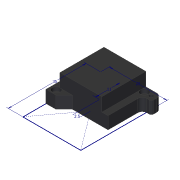
# Autodesk Inventor part: Raman2Go_Adapterplatte2_XY-TischChina
Saved by Autodesk Inventor 2019 (Build 230136000, 136)
## iProperties
Created: 2018-09-10
Part Number: Raman2Go_Adapterplatte2_XY-TischChina
Material: Generisch
Document SubType Name: Modeling
Designer: Henry John
Density: 1 g/cm^3
Appearance: Vorgabe
Author: Henry John
Autodesk Inventor part; units mm, degrees
ref_plane "YZ Plane" through (0, 0, 0) normal (1, 0, 0) x (0, 1, 0)
ref_plane "XZ Plane" through (0, 0, 0) normal (0, 1, 0) x (-1, 0, 0)
sketch "Skizze1" plane through (0, 0, 0) normal (0, 0, 1) x (1, 0, 0)
  line L0 (14.1792, -17.284) -> (14.1792, 17.716)
  line L1 (14.1792, 17.716) -> (-11.8208, 17.716)
  line L2 (-11.8208, 17.716) -> (-11.8208, -17.284)
  line L3 (-11.8208, -17.284) -> (14.1792, -17.284)
  line L4 (14.1792, -17.284) -> (-11.8208, 17.716) construction
  line L5 (14.1792, 17.716) -> (-11.8208, -17.284) construction
  line L6 (3.4292, 10.341) -> (-6.0708, 10.341) construction
  line L7 (3.4292, 3.091) -> (3.4292, 10.341) construction
  line L8 (-6.0708, 3.091) -> (3.4292, 3.091) construction
  line L9 (-6.0708, 10.341) -> (-6.0708, 3.091) construction
  line L10 (3.4292, 10.341) -> (-6.0708, 3.091) construction
  line L11 (3.4292, 3.091) -> (-6.0708, 10.341) construction
  point P0 (0, 0)
  point P1 (1.1792, 0.216)
  point P2 (1.1792, 0.216)
  point P3 (-1.3208, 6.716)
  point P4 (-1.3208, 6.716)
  point P5 (1.1792, 0.216)
  point P6 (-1.3208, 6.716)
  dimension "d0" = 26
  dimension "d1" = 35
  dimension "d2" = 11
  dimension "d3" = 2.5
  constraints: 16 end point, 6 midpoint, 2 parallel, 1 coincident, 1 perpendicular, 1 vertical
  measures "d0" distance of L1.end L0.end
  measures "d1" distance of L1.end L2.end
  measures "d2" distance from line of L1 point (-1.321, 6.716)
  measures "d3" horizontal distance of point (-1.321, 6.716) point (1.179, 0.216)
sketch "Skizze2" plane through (0, 0, 0) normal (0, 0, 1) x (1, 0, 0)
  line L0 (-3.4208, 1.091) -> (-7.8208, 1.091) projected
  line L1 (-7.8208, 1.091) -> (-7.8208, 12.341) projected
  line L2 (-7.8208, 12.341) -> (-3.4208, 12.341) projected
  line L3 (5.1792, 1.091) -> (0.7792, 1.091) projected
  line L4 (5.1792, 12.341) -> (5.1792, 1.091) projected
  line L5 (0.7792, 12.341) -> (5.1792, 12.341) projected
  circle A0 centre (-9.3002, -4.7384) radius 1.575 construction
  circle A1 centre (11.3792, 14.191) radius 1.575 construction
  circle A2 centre (-9.3002, -4.7384) radius 0.7 construction
  circle A3 centre (-10.7708, 16.016) radius 0.7 construction
  circle A4 centre (11.3792, 14.191) radius 0.7 construction
  line L6 (-3.4208, 12.341) -> (-3.4208, 13.366) projected
  line L7 (-3.4208, 13.366) -> (0.7792, 13.366) projected
  line L8 (0.7792, 0.066) -> (-3.4208, 0.066) projected
  line L9 (-3.4208, 0.066) -> (-3.4208, 1.091) projected
  line L10 (0.7792, 1.091) -> (0.7792, 0.066) projected
  line L11 (0.7792, 13.366) -> (0.7792, 12.341) projected
  line L12 (-12.2708, -9.259) -> (-12.2708, 10.741) construction
  line L13 (14.5292, 16.566) -> (-9.295, 16.566) construction
  arc A5 (16.5292, 14.566) -> (14.5292, 16.566) centre (14.5292, 14.566) ccw projected
  line L14 (16.5292, 14.566) -> (16.5292, 13.191) projected
  arc A6 (15.5292, 12.191) -> (16.5292, 13.191) centre (15.5292, 13.191) ccw projected
  line L15 (15.5292, 12.191) -> (14.4292, 12.191) projected
  arc A7 (14.4292, 12.191) -> (12.4292, 10.191) centre (14.4292, 10.191) ccw projected
  line L16 (12.4292, 10.191) -> (12.4292, -3.209) projected
  line L17 (-3.5708, -3.209) -> (12.4292, -3.209) projected
  line L18 (-8.1002, -7.7384) -> (-3.5708, -3.209) projected
  arc A8 (-10.7708, 17.591) -> (-9.295, 16.566) centre (-10.7708, 16.016) ccw construction
  line L19 (-8.1002, -8.7384) -> (-8.1002, -7.7384) construction
  circle A9 centre (-9.3002, -8.7384) radius 0.75 construction
  circle A10 centre (-9.3002, -8.7384) radius 1.2 construction
  line L20 (-10.8208, -7.909) -> (-11.8208, -6.909) construction
  line L21 (-11.8208, -6.909) -> (-11.8208, 14.7109)
  line L22 (-11.8208, -6.909) -> (-10.4976, -8.2322)
  arc A11 (-8.1002, -8.2384) -> (-8.2864, -7.9246) centre (-9.3002, -8.7384) ccw construction
  line L23 (-8.1002, -8.2384) -> (-8.1002, -7.7384) construction
  circle A12 centre (-9.3002, -4.7384) radius 1.675
  circle A13 centre (11.3792, 14.191) radius 1.675
  line L24 (14.5292, 16.566) -> (-9.1887, 16.566)
  arc A14 (-11.8208, 14.7109) -> (-9.1887, 16.566) centre (-10.7708, 16.016) ccw
  circle A15 centre (14.3792, 14.191) radius 0.75 construction
  circle A16 centre (14.3792, 14.191) radius 0.85
  line L25 (-8.1002, -7.7384) -> (-8.2864, -7.9246) construction
  arc A17 (-8.2864, -7.9246) -> (-10.4976, -8.2322) centre (-9.3002, -8.7384) ccw construction
  line L26 (-11.8208, -6.909) -> (-7.2708, -6.909)
  point P0 (0, 0)
  dimension "d4" = 0.1
  dimension "d5" = 0.1
  dimension "d6" = 0.1
  dimension "d7" = 0.1
  dimension "d10" = 0.1
  constraints: 12 end point, 6 centre point, 6 point on circle, 5 coincident, 3 point on line, 2 collinear, 1 horizontal, 1 vertical
  measures "d4" radial gap between concentric circles of A10 A11
  measures "d5" radial gap between concentric circles of A0 A12
  measures "d6" radial gap between concentric circles of A1 A13
  measures "d7" radial gap between concentric circles of A8 A14
  measures "d10" radial gap between concentric circles of A15 A16
extrude "Extrusion1" add sketch "Skizze2" along normal blind 2.5 contours L0 L1 L2 L6 L7 L11 L5 L4 L3 L10 L8 L9 | L14 A6 L15 A7 L16 L17 L18 L26 L21 A14 L24 A5
sketch "Skizze3" plane through (0, 0, 2.5) normal (0, 0, 1) x (1, 0, 0)
  circle A0 centre (11.3792, 14.191) radius 1.675 construction
  circle A1 centre (-9.3002, -4.7384) radius 1.675 construction
  circle A2 centre (14.3792, 14.191) radius 0.85 projected
  arc A3 (16.5292, 14.566) -> (14.5292, 16.566) centre (14.5292, 14.566) ccw projected
  line L0 (14.5292, 16.566) -> (-9.1887, 16.566) projected
  arc A4 (-11.8208, 14.7109) -> (-9.1887, 16.566) centre (-10.7708, 16.016) ccw construction
  line L1 (-11.8208, 14.7109) -> (-11.8208, -6.909) projected
  line L2 (-7.2708, -6.909) -> (-3.5708, -3.209) projected
  line L3 (-3.5708, -3.209) -> (12.4292, -3.209) projected
  line L4 (12.4292, -3.209) -> (12.4292, 10.191) projected
  arc A5 (14.4292, 12.191) -> (12.4292, 10.191) centre (14.4292, 10.191) ccw projected
  line L5 (14.4292, 12.191) -> (15.5292, 12.191) projected
  arc A6 (15.5292, 12.191) -> (16.5292, 13.191) centre (15.5292, 13.191) ccw projected
  line L6 (16.5292, 13.191) -> (16.5292, 14.566) projected
  circle A7 centre (11.3792, 14.191) radius 0.7 construction
  circle A8 centre (-9.3002, -4.7384) radius 0.7 construction
  circle A9 centre (-9.3002, -8.7384) radius 0.75 construction
  circle A10 centre (-9.3002, -8.7384) radius 0.85
  line L7 (-8.2864, -7.9246) -> (-3.5708, -3.209) projected
  arc A11 (-10.4976, -8.2322) -> (-8.2864, -7.9246) centre (-9.3002, -8.7384) ccw
  arc A12 (-9.1887, 16.566) -> (-11.8208, 14.7109) centre (-10.7708, 16.016) ccw
  circle A13 centre (-10.7708, 16.016) radius 0.7 construction
  circle A14 centre (-10.7708, 16.016) radius 0.9
  circle A15 centre (11.3792, 14.191) radius 0.9
  circle A16 centre (-9.3002, -4.7384) radius 0.9
  line L8 (-11.8208, -6.909) -> (-7.2708, -6.909) projected
  point P0 (0, 0)
  dimension "d11" = 0.1
  dimension "d13" = 1.8
  dimension "d14" = 1.8
  dimension "d15" = 1.8
  constraints: 6 centre point, 6 coincident, 4 point on circle
  measures "d11" radial gap between concentric circles of A9 A10
  measures "d13" diameter of A14
  measures "d14" diameter of A15
  measures "d15" diameter of A16
ref_plane "Arbeitsebene1" through (-9.7716, -9.2098, 6) normal (0, 0, 1) x (1, 0, 0)
extrude "Extrusion2" add sketch "Skizze3" along normal blind 3 contours L6 A6 L5 A5 L4 L3 L2 L8 L1 A12 L0 A3
sketch "Skizze4" plane through (-9.1887, 16.566, 5.5) normal (0, 0, 1) x (1, 0, 0)
  circle A0 centre (-0.1115, -21.3043) radius 0.7 construction
  circle A1 centre (-1.5821, -0.55) radius 0.7 construction
  circle A2 centre (20.5679, -2.375) radius 0.7 construction
  point P0 (9.1887, -16.566)
hole "Bohrung1" at (-9.3002, -4.7384, 5.5) at (11.3792, 14.191, 5.5) direction (0, 0, -1) diameter 1.8 end through all counterbore diameter 3.5 counterbore depth 1.8 clearance for "Inbusschraube ISO 4762" size "M1.6" standard "ISO"
sketch "Sketch8" plane through (0, 0, 5.5) normal (0, 0, 1) x (1, 0, 0)
  circle A0 centre (-9.3002, -4.7384) radius 1.75 projected
  circle A1 centre (11.3792, 14.191) radius 1.75 projected
  circle A2 centre (-10.7708, 16.016) radius 0.9 projected
  circle A3 centre (14.3792, 14.191) radius 0.85 projected
  arc A4 (16.5292, 14.566) -> (14.5292, 16.566) centre (14.5292, 14.566) ccw projected
  line L0 (14.5292, 16.566) -> (-9.1887, 16.566) projected
  arc A5 (-9.1887, 16.566) -> (-11.8208, 14.7109) centre (-10.7708, 16.016) ccw projected
  line L1 (-11.8208, 14.7109) -> (-11.8208, -6.909) projected
  line L2 (-11.8208, -6.909) -> (-7.2708, -6.909) projected
  line L3 (-7.2708, -6.909) -> (-3.5708, -3.209) projected
  line L4 (-3.5708, -3.209) -> (12.4292, -3.209) projected
  line L5 (12.4292, -3.209) -> (12.4292, 10.191) projected
  arc A6 (14.4292, 12.191) -> (12.4292, 10.191) centre (14.4292, 10.191) ccw projected
  line L6 (14.4292, 12.191) -> (15.5292, 12.191) projected
  arc A7 (15.5292, 12.191) -> (16.5292, 13.191) centre (15.5292, 13.191) ccw projected
  line L7 (16.5292, 13.191) -> (16.5292, 14.566) projected
  line L8 (12.4292, -3.209) -> (-3.5708, -3.209) projected
  line L9 (-9.1887, 16.566) -> (14.5292, 16.566) projected
  line L10 (9.6292, -3.209) -> (-9.1887, -3.209)
  line L11 (-9.1887, -3.209) -> (-9.1887, 16.566)
  line L12 (-9.1887, 16.566) -> (9.6292, 16.566)
  line L13 (9.6292, 16.566) -> (9.6292, -3.209)
  circle A8 centre (11.3792, 14.191) radius 1.75 projected
  point P0 (0, 0)
  constraints: 8 end point, 2 parallel, 1 horizontal, 1 perpendicular, 1 point on line, 1 tangent
extrude "Extrusion6" add sketch "Sketch8" along normal blind 6 contours L10 L11 A0 | A0 L11 L0 L13 L4 L10 picked at (-8.7742, -3.1728)
